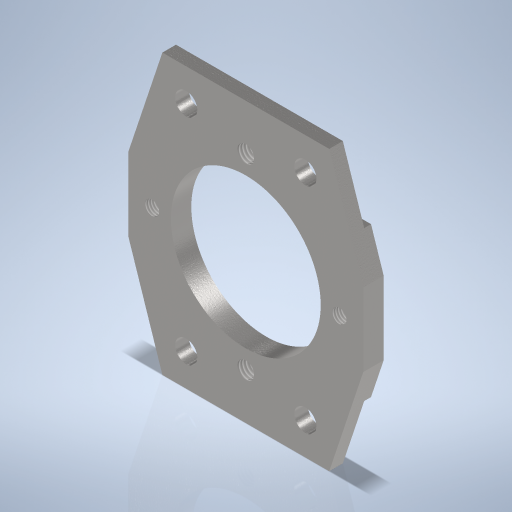
# Autodesk Inventor part: HAlteplatte
Saved by Autodesk Inventor 2024 (Build 280153000, 153)
## iProperties
Created: 2024-03-01
Part Number: HAlteplatte
Material: Stahl, galvanisiert
Document SubType Name: Modeling
Designer: ffogue
Density: 7.85 g/cm^3
Appearance: Galvanisiert
Author: ffogue
Autodesk Inventor part; units mm, degrees
ref_plane "YZ Plane" through (0, 0, 0) normal (1, 0, 0) x (0, 1, 0)
ref_plane "XZ Plane" through (0, 0, 0) normal (0, 1, 0) x (-1, 0, 0)
sketch "Skizze1" plane through (0, 0, 0) normal (0, 1, 0) x (-1, 0, 0)
  line L0 (0, 10.7628) -> (10, 41)
  line L1 (10, 41) -> (59, 41)
  line L2 (59, 41) -> (69, 10.7628)
  line L3 (69, 10.7628) -> (69, -10.7628)
  line L4 (69, -10.7628) -> (59, -41)
  line L5 (59, -41) -> (10, -41)
  line L6 (10, -41) -> (0, -10.7628)
  line L7 (0, -10.7628) -> (0, 10.7628)
  line L8 (34.5, 41) -> (34.5, -41) construction
  line L9 (0, 0) -> (92.3843, 0) construction
  dimension "d0" = 69
  dimension "d1" = 18.3
  dimension "d2" = 49
  dimension "d4" = 82
  dimension "d5" = 18.3
  dimension "d6" = 18.3
  dimension "d7" = 18.3
  constraints: 20 end point, 3 midpoint, 2 horizontal, 2 horizontal alignment, 2 parallel, 2 perpendicular, 1 coincident, 1 point on line, 1 vertical alignment
  measures "d0" distance between parallel lines of L7 L3
  measures "d1" angle of L0 L7
  measures "d2" distance of L4.end L5.end
  measures "d4" distance between parallel lines of L5 L1
  measures "d5" angle of L6 L7
  measures "d6" angle of L2 L3
  measures "d7" angle of L4 L3
extrude "Extrusion1" add sketch "Skizze1" along normal blind 4
sketch "Skizze2" plane through (0, 4, 0) normal (0, 1, 0) x (1, 0, 0)
  line L0 (-69, -10.7628) -> (-59, -41) projected
  line L1 (-65.2836, -22) -> (-3.7164, -22)
  line L2 (-59, -41) -> (-10, -41) projected
  line L3 (-59, 41) -> (-69, 10.7628) projected
  line L4 (-65.2836, 22) -> (-3.7164, 22)
  line L5 (0, 10.7628) -> (-10, 41) projected
  line L6 (0, 0) -> (-69, 0) construction
  line L7 (-69, 10.7628) -> (-69, -10.7628) projected
  line L8 (0, -10.7628) -> (0, 10.7628) projected
  line L9 (-10, -41) -> (0, -10.7628) projected
  dimension "d10" = 44
  constraints: 6 end point, 3 point on line, 2 horizontal, 2 vertical alignment, 1 parallel, 1 other
  measures "d10" distance between parallel lines of L4 L1
extrude "Extrusion2" add sketch "Skizze2" along normal blind 2 contours L7 L3 L4 L5 L8 L9 L1 L0
sketch "Skizze3" plane through (0, 6, 0) normal (0, 1, 0) x (1, 0, 0)
  circle A0 centre (-34.5, 0) radius 22
  line L0 (0, -10.7628) -> (0, 10.7628) projected
  line L1 (-59, -41) -> (-10, -41) projected
  point P0 (0, 0)
  point P1 (0, 0)
  point P2 (-34.5, -41)
  dimension "d13" = 44
  constraints: 2 midpoint, 1 centre point, 1 horizontal alignment, 1 vertical alignment
  measures "d13" diameter of A0
extrude "Extrusion3" cut sketch "Skizze3" against normal up to surface (6 mm away)
sketch "Skizze4" plane through (0, 4, 0) normal (0, 1, 0) x (1, 0, 0)
  line L0 (-10, 41) -> (-59, 41) projected
  line L1 (0, 0) -> (-69, 0) construction
  line L2 (-69, 10.7628) -> (-69, -10.7628) projected
  point P0 (-34.5, 27.5)
  point P1 (-34.5, -27.5)
  point P2 (-34.5, 41)
  dimension "d16" = 55
  constraints: 2 end point, 2 midpoint, 1 symmetric about line, 1 vertical alignment
  measures "d16" distance of point (-34.5, -27.5) point (-34.5, 27.5)
hole "Bohrung1" at (-34.5, 4, -27.5) at (-34.5, 4, 27.5) direction (0, -1, 0) diameter 4.917 end through all thread size "M6x1" class "6H" standard "ISO Metric profile"
sketch "Skizze5" plane through (0, 4, 0) normal (0, 1, 0) x (1, 0, 0)
  line L0 (-10, 41) -> (-59, 41) projected
  line L1 (-34.5, 41) -> (-34.5, 22) construction
  line L2 (0, 0) -> (-76.2503, 0) construction
  point P0 (-17, 31.5)
  point P1 (-52, 31.5)
  point P2 (-34.5, 31.5)
  point P3 (-17, -31.5)
  point P4 (-52, -31.5)
  dimension "d31" = 35
  dimension "d42" = 35
  dimension "d43" = 63
  constraints: 4 end point, 2 horizontal alignment, 2 midpoint, 2 symmetric about line, 2 vertical alignment, 1 horizontal, 1 vertical
  measures "d31" distance of point (-52, 31.5) point (-17, 31.5)
  measures "d42" distance of point (-17, -31.5) point (-52, -31.5)
  measures "d43" distance of point (-17, -31.5) point (-17, 31.5)
hole "Bohrung2" at (-17, 4, -31.5) at (-52, 4, -31.5) at (-17, 4, 31.5) at (-52, 4, 31.5) direction (0, -1, 0) diameter 6.5 end through all
sketch "Skizze6" plane through (0, 6, 0) normal (0, 1, 0) x (1, 0, 0)
  line L0 (0, -10.7628) -> (0, 10.7628) projected
  line L1 (-10, 41) -> (-59, 41) projected
  line L2 (-34.5, 41) -> (-34.5, -41) construction
  line L3 (-59, -41) -> (-10, -41) projected
  point P0 (0, 0)
  point P1 (-7, 0)
  point P2 (-62, 0)
  point P3 (0, 0)
  point P4 (0, 0)
  dimension "d33" = 55
  constraints: 4 midpoint, 2 end point, 2 horizontal alignment, 1 symmetric about line
  measures "d33" distance of point (-62, 0) point (-7, 0)
hole "Bohrung3" at (-7, 6, 0) at (-62, 6, 0) direction (0, -1, 0) diameter 4.134 end through all thread size "M5x0.8" class "6H" standard "ISO Metric profile"
ref_plane "Arbeitsebene1" through (-10, 0, 0) normal (0, 0, -1) x (-1, 0, 0)
equation "\"d5\" = d1"
equation "\"d6\" = d1"
equation "\"d7\" = d6"
